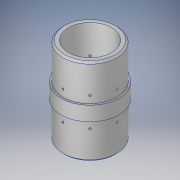
# Autodesk Inventor part: section_adapter
Saved by Autodesk Inventor 2017 SP1 (Build 210196100, 196)
## iProperties
Created: 2016-10-29
Part Number: section_adapter
Material: Aluminum 6061
Document SubType Name: Modeling
Designer: cflannery
Density: 2.7 g/cm^3
Appearance: Aluminum - Flat
Author: cflannery
Autodesk Inventor part; units mm, degrees
ref_plane "YZ Plane" through (0, 0, 0) normal (1, 0, 0) x (0, 1, 0)
ref_plane "XZ Plane" through (0, 0, 0) normal (0, 1, 0) x (-1, 0, 0)
sketch "Sketch1" plane through (0, 0, 0) normal (0, 1, 0) x (-1, 0, 0)
  circle A0 centre (0, 0) radius 101.6
  circle A1 centre (0, 0) radius 50.8
  dimension "d0" = 203.2
  dimension "d1" = 101.6
  constraints: 2 centre point, 2 coincident
  measures "d0" diameter of A0
  measures "d1" diameter of A1
extrude "Extrusion1" add sketch "Sketch1" along normal mid plane 50.8
sketch "Sketch2" plane through (0, 25.4, 0) normal (0, 1, 0) x (1, 0, 0)
  circle A0 centre (0, 0) radius 95.25
  circle A1 centre (0, 0) radius 76.2
  dimension "d4" = 190.5
  dimension "d5" = 152.4
  constraints: 2 centre point, 2 coincident
  measures "d4" diameter of A0
  measures "d5" diameter of A1
extrude "Extrusion2" add sketch "Sketch2" along normal blind 127
sketch "Sketch3" plane through (0, -25.4, 0) normal (0, -1, 0) x (1, 0, 0)
  circle A0 centre (0, 0) radius 95.25
  circle A1 centre (0, 0) radius 76.2
  dimension "d8" = 152.4
  dimension "d9" = 190.5
  constraints: 2 centre point, 2 coincident
  measures "d8" diameter of A1
  measures "d9" diameter of A0
extrude "Extrusion3" add sketch "Sketch3" along normal blind 127
ref_plane "Work Plane1" through (0, -25.4, -95.25) normal (0, 0, 1) x (1, 0, 0)
sketch "Sketch4" plane through (0, -25.4, -95.25) normal (0, 0, 1) x (1, 0, 0)
  line L0 (101.6, 50.8) -> (-101.6, 50.8) projected
  line L1 (-101.6, 0) -> (101.6, 0) projected
  point P0 (0, 25.4)
  point P1 (0, -25.4)
  point P2 (0, 76.2)
  dimension "d12" = 25.4
  dimension "d13" = 25.4
  measures "d12" distance from line of L0 point (0, 76.2)
  measures "d13" distance from line of L1 point (0, -25.4)
hole "Hole1" at (0, -50.8, -95.25) at (0, 50.8, -95.25) direction (0, 0, 1) diameter 6.35 depth 25.4 tip angle 118
pattern_circular "Circular Pattern1" count 8 over 360 about axis through (0, -25.4, 0) along (0, -1, 0) of "Hole1"
chamfer "Chamfer1" distance 6.35 angle 45 2 edges at (-95.25, -152.4, 0) (-95.25, 152.4, 0)
body "Solid1"
